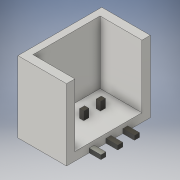
# Autodesk Inventor part: RZ_3Pos_1mm_SM_Header
Saved by Autodesk Inventor 2016 (Build 200138000, 138)
## iProperties
Created: 2016-09-14
Part Number: RZ_3Pos_1mm_SM_Header
Material: Generic
Document SubType Name: Modeling
Designer: jfixelle
Density: 1 g/cm^3
Appearance: White
Author: jfixelle
Autodesk Inventor part; units mm, degrees
ref_plane "YZ Plane" through (0, 0, 0) normal (1, 0, 0) x (0, 1, 0)
ref_plane "XZ Plane" through (0, 0, 0) normal (0, 1, 0) x (-1, 0, 0)
ref_plane "XY Plane" through (0, 0, 0) normal (0, 0, 1) x (1, 0, 0)
sketch "Sketch1" plane through (0, 0, 0) normal (0, 1, 0) x (-1, 0, 0)
  line L0 (1.45, 2.5) -> (-1.45, 2.5)
  line L1 (-1.45, 2.5) -> (-1.45, -2.5)
  line L2 (-1.45, -2.5) -> (1.45, -2.5)
  line L3 (1.45, -2.5) -> (1.45, 2.5)
  point P0 (0, 0)
  dimension "d0" = 2.9
  dimension "d1" = 1.45
  dimension "d2" = 5
  dimension "d3" = 2.5
  constraints: 8 end point, 2 parallel, 1 horizontal, 1 perpendicular
  measures "d0" distance of L1.end L2.end
  measures "d1" distance from line of point (0, 0) L3
  measures "d2" distance of L2.end L0.start
  measures "d3" distance from line of L2 point (0, 0)
extrude "Extrusion1" add sketch "Sketch1" along normal blind 4.25
sketch "Sketch2" plane through (0, 4.25, 0) normal (0, 1, 0) x (1, 0, 0)
  line L0 (1.45, -2.5) -> (1.45, 2.5) projected
  line L1 (1.45, -2) -> (-1.05, -2)
  line L2 (-1.05, -2) -> (-1.05, 2)
  line L3 (-1.05, 2) -> (1.45, 2)
  line L4 (1.45, 2) -> (1.45, -2)
  point P0 (0, 0)
  dimension "d6" = 4
  dimension "d7" = 2
  dimension "d8" = 2.5
  constraints: 8 end point, 2 parallel, 1 horizontal, 1 perpendicular, 1 point on line
  measures "d6" distance of L1.end L2.end
  measures "d7" distance from line of point (0, 0) L3
  measures "d8" distance of L1.start L1.end
extrude "Extrusion2" cut sketch "Sketch2" against normal blind 3.75
sketch "Sketch3" plane through (0, 0, 0) normal (0, 0, 1) x (1, 0, 0)
  line L0 (0.125, 1) -> (-0.125, 1)
  line L1 (-0.125, 1) -> (-0.125, 0)
  line L2 (-0.125, 0) -> (2.15, 0)
  line L3 (2.15, 0) -> (2.15, 0.25)
  line L4 (2.15, 0.25) -> (0.125, 0.25)
  line L5 (0.125, 0.25) -> (0.125, 1)
  point P0 (0, 0)
  dimension "d11" = 2.15
  dimension "d12" = 0
  dimension "d13" = 0.25
  dimension "d14" = 0.25
  dimension "d15" = 0.125
  dimension "d16" = 1
  constraints: 12 end point, 5 perpendicular, 1 horizontal
  measures "d11" distance from line of point (0, 0) L3
  measures "d12" distance from line of L2 point (0, 0)
  measures "d13" distance of L2.end L3.end
  measures "d14" distance of L0.start L0.end
  measures "d15" distance from line of L1 point (0, 0)
  measures "d16" distance of L0.end L1.end
extrude "Extrusion3" add sketch "Sketch3" along normal mid plane 0.3
pattern_linear "Rectangular Pattern1" count 3 spacing 1 along (0, 0, 1) of "Extrusion3" first direction both ways yes
body "Solid1"
